Autodesk Inventor part; units mm, degrees
(part 7 of 15)
  arc A2930 (57.5832, 42.092) -> (57.6848, 42.092) centre (57.634, 42.092) ccw
  line L1321 (60.642, 43.084) -> (60.642, 45.116)
  arc A2931 (60.6928, 45.116) -> (60.5912, 45.116) centre (60.642, 45.116) ccw
  arc A2932 (60.5912, 43.084) -> (60.6928, 43.084) centre (60.642, 43.084) ccw
  line L1322 (60.642, 45.116) -> (61.658, 45.116)
  arc A2933 (61.658, 45.0652) -> (61.658, 45.1668) centre (61.658, 45.116) ccw
  arc A2934 (60.642, 45.1668) -> (60.642, 45.0652) centre (60.642, 45.116) ccw
  line L1323 (61.658, 45.116) -> (61.658, 43.084)
  arc A2935 (61.6072, 43.084) -> (61.7088, 43.084) centre (61.658, 43.084) ccw
  arc A2936 (61.7088, 45.116) -> (61.6072, 45.116) centre (61.658, 45.116) ccw
  line L1324 (61.658, 43.084) -> (60.642, 43.084)
  arc A2937 (60.642, 43.1348) -> (60.642, 43.0332) centre (60.642, 43.084) ccw
  arc A2938 (61.658, 43.0332) -> (61.658, 43.1348) centre (61.658, 43.084) ccw
  line L1325 (55.658, 51.116) -> (55.658, 49.084)
  arc A2939 (55.6072, 49.084) -> (55.7088, 49.084) centre (55.658, 49.084) ccw
  arc A2940 (55.7088, 51.116) -> (55.6072, 51.116) centre (55.658, 51.116) ccw
  line L1326 (55.658, 49.084) -> (54.642, 49.084)
  arc A2941 (54.642, 49.1348) -> (54.642, 49.0332) centre (54.642, 49.084) ccw
  arc A2942 (55.658, 49.0332) -> (55.658, 49.1348) centre (55.658, 49.084) ccw
  line L1327 (54.642, 49.084) -> (54.642, 51.116)
  arc A2943 (54.6928, 51.116) -> (54.5912, 51.116) centre (54.642, 51.116) ccw
  arc A2944 (54.5912, 49.084) -> (54.6928, 49.084) centre (54.642, 49.084) ccw
  line L1328 (54.642, 51.116) -> (55.658, 51.116)
  arc A2945 (55.658, 51.0652) -> (55.658, 51.1668) centre (55.658, 51.116) ccw
  arc A2946 (54.642, 51.1668) -> (54.642, 51.0652) centre (54.642, 51.116) ccw
  line L1329 (61.166, 33.892) -> (59.134, 33.892)
  arc A2947 (59.134, 33.9428) -> (59.134, 33.8412) centre (59.134, 33.892) ccw
  arc A2948 (61.166, 33.8412) -> (61.166, 33.9428) centre (61.166, 33.892) ccw
  line L1330 (59.134, 33.892) -> (59.134, 34.908)
  arc A2949 (59.1848, 34.908) -> (59.0832, 34.908) centre (59.134, 34.908) ccw
  arc A2950 (59.0832, 33.892) -> (59.1848, 33.892) centre (59.134, 33.892) ccw
  line L1331 (59.134, 34.908) -> (61.166, 34.908)
  arc A2951 (61.166, 34.8572) -> (61.166, 34.9588) centre (61.166, 34.908) ccw
  arc A2952 (59.134, 34.9588) -> (59.134, 34.8572) centre (59.134, 34.908) ccw
  line L1332 (61.166, 34.908) -> (61.166, 33.892)
  arc A2953 (61.1152, 33.892) -> (61.2168, 33.892) centre (61.166, 33.892) ccw
  arc A2954 (61.2168, 34.908) -> (61.1152, 34.908) centre (61.166, 34.908) ccw
  line L1333 (63.166, 33.892) -> (61.134, 33.892)
  arc A2955 (61.134, 33.9428) -> (61.134, 33.8412) centre (61.134, 33.892) ccw
  arc A2956 (63.166, 33.8412) -> (63.166, 33.9428) centre (63.166, 33.892) ccw
  line L1334 (61.134, 33.892) -> (61.134, 34.908)
  arc A2957 (61.1848, 34.908) -> (61.0832, 34.908) centre (61.134, 34.908) ccw
  arc A2958 (61.0832, 33.892) -> (61.1848, 33.892) centre (61.134, 33.892) ccw
  line L1335 (61.134, 34.908) -> (63.166, 34.908)
  arc A2959 (63.166, 34.8572) -> (63.166, 34.9588) centre (63.166, 34.908) ccw
  arc A2960 (61.134, 34.9588) -> (61.134, 34.8572) centre (61.134, 34.908) ccw
  line L1336 (63.166, 34.908) -> (63.166, 33.892)
  arc A2961 (63.1152, 33.892) -> (63.2168, 33.892) centre (63.166, 33.892) ccw
  arc A2962 (63.2168, 34.908) -> (63.1152, 34.908) centre (63.166, 34.908) ccw
  line L1337 (52.658, 43.116) -> (52.658, 41.084)
  arc A2963 (52.6072, 41.084) -> (52.7088, 41.084) centre (52.658, 41.084) ccw
  arc A2964 (52.7088, 43.116) -> (52.6072, 43.116) centre (52.658, 43.116) ccw
  line L1338 (52.658, 41.084) -> (51.642, 41.084)
  arc A2965 (51.642, 41.1348) -> (51.642, 41.0332) centre (51.642, 41.084) ccw
  arc A2966 (52.658, 41.0332) -> (52.658, 41.1348) centre (52.658, 41.084) ccw
  line L1339 (51.642, 41.084) -> (51.642, 43.116)
  arc A2967 (51.6928, 43.116) -> (51.5912, 43.116) centre (51.642, 43.116) ccw
  arc A2968 (51.5912, 41.084) -> (51.6928, 41.084) centre (51.642, 41.084) ccw
  line L1340 (51.642, 43.116) -> (52.658, 43.116)
  arc A2969 (52.658, 43.0652) -> (52.658, 43.1668) centre (52.658, 43.116) ccw
  arc A2970 (51.642, 43.1668) -> (51.642, 43.0652) centre (51.642, 43.116) ccw
  line L1341 (51.666, 42.092) -> (49.634, 42.092)
  arc A2971 (49.634, 42.1428) -> (49.634, 42.0412) centre (49.634, 42.092) ccw
  arc A2972 (51.666, 42.0412) -> (51.666, 42.1428) centre (51.666, 42.092) ccw
  line L1342 (49.634, 42.092) -> (49.634, 43.108)
  arc A2973 (49.6848, 43.108) -> (49.5832, 43.108) centre (49.634, 43.108) ccw
  arc A2974 (49.5832, 42.092) -> (49.6848, 42.092) centre (49.634, 42.092) ccw
  line L1343 (49.634, 43.108) -> (51.666, 43.108)
  arc A2975 (51.666, 43.0572) -> (51.666, 43.1588) centre (51.666, 43.108) ccw
  arc A2976 (49.634, 43.1588) -> (49.634, 43.0572) centre (49.634, 43.108) ccw
  line L1344 (51.666, 43.108) -> (51.666, 42.092)
  arc A2977 (51.6152, 42.092) -> (51.7168, 42.092) centre (51.666, 42.092) ccw
  arc A2978 (51.7168, 43.108) -> (51.6152, 43.108) centre (51.666, 43.108) ccw
  line L1345 (51.634, 49.108) -> (53.666, 49.108)
  arc A2979 (53.666, 49.0572) -> (53.666, 49.1588) centre (53.666, 49.108) ccw
  arc A2980 (51.634, 49.1588) -> (51.634, 49.0572) centre (51.634, 49.108) ccw
  line L1346 (53.666, 49.108) -> (53.666, 48.092)
  arc A2981 (53.6152, 48.092) -> (53.7168, 48.092) centre (53.666, 48.092) ccw
  arc A2982 (53.7168, 49.108) -> (53.6152, 49.108) centre (53.666, 49.108) ccw
  line L1347 (53.666, 48.092) -> (51.634, 48.092)
  arc A2983 (51.634, 48.1428) -> (51.634, 48.0412) centre (51.634, 48.092) ccw
  arc A2984 (53.666, 48.0412) -> (53.666, 48.1428) centre (53.666, 48.092) ccw
  line L1348 (51.634, 48.092) -> (51.634, 49.108)
  arc A2985 (51.6848, 49.108) -> (51.5832, 49.108) centre (51.634, 49.108) ccw
  arc A2986 (51.5832, 48.092) -> (51.6848, 48.092) centre (51.634, 48.092) ccw
  line L1349 (51.634, 44.108) -> (53.666, 44.108)
  arc A2987 (53.666, 44.0572) -> (53.666, 44.1588) centre (53.666, 44.108) ccw
  arc A2988 (51.634, 44.1588) -> (51.634, 44.0572) centre (51.634, 44.108) ccw
  line L1350 (53.666, 44.108) -> (53.666, 43.092)
  arc A2989 (53.6152, 43.092) -> (53.7168, 43.092) centre (53.666, 43.092) ccw
  arc A2990 (53.7168, 44.108) -> (53.6152, 44.108) centre (53.666, 44.108) ccw
  line L1351 (53.666, 43.092) -> (51.634, 43.092)
  arc A2991 (51.634, 43.1428) -> (51.634, 43.0412) centre (51.634, 43.092) ccw
  arc A2992 (53.666, 43.0412) -> (53.666, 43.1428) centre (53.666, 43.092) ccw
  line L1352 (51.634, 43.092) -> (51.634, 44.108)
  arc A2993 (51.6848, 44.108) -> (51.5832, 44.108) centre (51.634, 44.108) ccw
  arc A2994 (51.5832, 43.092) -> (51.6848, 43.092) centre (51.634, 43.092) ccw
  line L1353 (51.634, 45.108) -> (53.666, 45.108)
  arc A2995 (53.666, 45.0572) -> (53.666, 45.1588) centre (53.666, 45.108) ccw
  arc A2996 (51.634, 45.1588) -> (51.634, 45.0572) centre (51.634, 45.108) ccw
  line L1354 (53.666, 45.108) -> (53.666, 44.092)
  arc A2997 (53.6152, 44.092) -> (53.7168, 44.092) centre (53.666, 44.092) ccw
  arc A2998 (53.7168, 45.108) -> (53.6152, 45.108) centre (53.666, 45.108) ccw
  line L1355 (53.666, 44.092) -> (51.634, 44.092)
  arc A2999 (51.634, 44.1428) -> (51.634, 44.0412) centre (51.634, 44.092) ccw
  arc A3000 (53.666, 44.0412) -> (53.666, 44.1428) centre (53.666, 44.092) ccw
  line L1356 (51.634, 44.092) -> (51.634, 45.108)
  arc A3001 (51.6848, 45.108) -> (51.5832, 45.108) centre (51.634, 45.108) ccw
  arc A3002 (51.5832, 44.092) -> (51.6848, 44.092) centre (51.634, 44.092) ccw
  line L1357 (67.958, 53.716) -> (67.958, 51.684)
  arc A3003 (67.9072, 51.684) -> (68.0088, 51.684) centre (67.958, 51.684) ccw
  arc A3004 (68.0088, 53.716) -> (67.9072, 53.716) centre (67.958, 53.716) ccw
  line L1358 (67.958, 51.684) -> (66.942, 51.684)
  arc A3005 (66.942, 51.7348) -> (66.942, 51.6332) centre (66.942, 51.684) ccw
  arc A3006 (67.958, 51.6332) -> (67.958, 51.7348) centre (67.958, 51.684) ccw
  line L1359 (66.942, 51.684) -> (66.942, 53.716)
  arc A3007 (66.9928, 53.716) -> (66.8912, 53.716) centre (66.942, 53.716) ccw
  arc A3008 (66.8912, 51.684) -> (66.9928, 51.684) centre (66.942, 51.684) ccw
  line L1360 (66.942, 53.716) -> (67.958, 53.716)
  arc A3009 (67.958, 53.6652) -> (67.958, 53.7668) centre (67.958, 53.716) ccw
  arc A3010 (66.942, 53.7668) -> (66.942, 53.6652) centre (66.942, 53.716) ccw
  line L1361 (61.442, 51.684) -> (61.442, 53.716)
  arc A3011 (61.4928, 53.716) -> (61.3912, 53.716) centre (61.442, 53.716) ccw
  arc A3012 (61.3912, 51.684) -> (61.4928, 51.684) centre (61.442, 51.684) ccw
  line L1362 (61.442, 53.716) -> (62.458, 53.716)
  arc A3013 (62.458, 53.6652) -> (62.458, 53.7668) centre (62.458, 53.716) ccw
  arc A3014 (61.442, 53.7668) -> (61.442, 53.6652) centre (61.442, 53.716) ccw
  line L1363 (62.458, 53.716) -> (62.458, 51.684)
  arc A3015 (62.4072, 51.684) -> (62.5088, 51.684) centre (62.458, 51.684) ccw
  arc A3016 (62.5088, 53.716) -> (62.4072, 53.716) centre (62.458, 53.716) ccw
  line L1364 (62.458, 51.684) -> (61.442, 51.684)
  arc A3017 (61.442, 51.7348) -> (61.442, 51.6332) centre (61.442, 51.684) ccw
  arc A3018 (62.458, 51.6332) -> (62.458, 51.7348) centre (62.458, 51.684) ccw
  line L1365 (-2.616, 56.708) -> (-0.584, 56.708)
  arc A3019 (-0.584, 56.6572) -> (-0.584, 56.7588) centre (-0.584, 56.708) ccw
  arc A3020 (-2.616, 56.7588) -> (-2.616, 56.6572) centre (-2.616, 56.708) ccw
  line L1366 (-0.584, 56.708) -> (-0.584, 55.692)
  arc A3021 (-0.6348, 55.692) -> (-0.5332, 55.692) centre (-0.584, 55.692) ccw
  arc A3022 (-0.5332, 56.708) -> (-0.6348, 56.708) centre (-0.584, 56.708) ccw
  line L1367 (-0.584, 55.692) -> (-2.616, 55.692)
  arc A3023 (-2.616, 55.7428) -> (-2.616, 55.6412) centre (-2.616, 55.692) ccw
  arc A3024 (-0.584, 55.6412) -> (-0.584, 55.7428) centre (-0.584, 55.692) ccw
  line L1368 (-2.616, 55.692) -> (-2.616, 56.708)
  arc A3025 (-2.5652, 56.708) -> (-2.6668, 56.708) centre (-2.616, 56.708) ccw
  arc A3026 (-2.6668, 55.692) -> (-2.5652, 55.692) centre (-2.616, 55.692) ccw
  line L1369 (-0.584, 51.692) -> (-2.616, 51.692)
  arc A3027 (-2.616, 51.7428) -> (-2.616, 51.6412) centre (-2.616, 51.692) ccw
  arc A3028 (-0.584, 51.6412) -> (-0.584, 51.7428) centre (-0.584, 51.692) ccw
  line L1370 (-2.616, 51.692) -> (-2.616, 52.708)
  arc A3029 (-2.5652, 52.708) -> (-2.6668, 52.708) centre (-2.616, 52.708) ccw
  arc A3030 (-2.6668, 51.692) -> (-2.5652, 51.692) centre (-2.616, 51.692) ccw
  line L1371 (-2.616, 52.708) -> (-0.584, 52.708)
  arc A3031 (-0.584, 52.6572) -> (-0.584, 52.7588) centre (-0.584, 52.708) ccw
  arc A3032 (-2.616, 52.7588) -> (-2.616, 52.6572) centre (-2.616, 52.708) ccw
  line L1372 (-0.584, 52.708) -> (-0.584, 51.692)
  arc A3033 (-0.6348, 51.692) -> (-0.5332, 51.692) centre (-0.584, 51.692) ccw
  arc A3034 (-0.5332, 52.708) -> (-0.6348, 52.708) centre (-0.584, 52.708) ccw
  line L1373 (-2.616, 53.708) -> (-0.584, 53.708)
  arc A3035 (-0.584, 53.6572) -> (-0.584, 53.7588) centre (-0.584, 53.708) ccw
  arc A3036 (-2.616, 53.7588) -> (-2.616, 53.6572) centre (-2.616, 53.708) ccw
  line L1374 (-0.584, 53.708) -> (-0.584, 52.692)
  arc A3037 (-0.6348, 52.692) -> (-0.5332, 52.692) centre (-0.584, 52.692) ccw
  arc A3038 (-0.5332, 53.708) -> (-0.6348, 53.708) centre (-0.584, 53.708) ccw
  line L1375 (-0.584, 52.692) -> (-2.616, 52.692)
  arc A3039 (-2.616, 52.7428) -> (-2.616, 52.6412) centre (-2.616, 52.692) ccw
  arc A3040 (-0.584, 52.6412) -> (-0.584, 52.7428) centre (-0.584, 52.692) ccw
  line L1376 (-2.616, 52.692) -> (-2.616, 53.708)
  arc A3041 (-2.5652, 53.708) -> (-2.6668, 53.708) centre (-2.616, 53.708) ccw
  arc A3042 (-2.6668, 52.692) -> (-2.5652, 52.692) centre (-2.616, 52.692) ccw
  line L1377 (-2.616, 54.708) -> (-0.584, 54.708)
  arc A3043 (-0.584, 54.6572) -> (-0.584, 54.7588) centre (-0.584, 54.708) ccw
  arc A3044 (-2.616, 54.7588) -> (-2.616, 54.6572) centre (-2.616, 54.708) ccw
  line L1378 (-0.584, 54.708) -> (-0.584, 53.692)
  arc A3045 (-0.6348, 53.692) -> (-0.5332, 53.692) centre (-0.584, 53.692) ccw
  arc A3046 (-0.5332, 54.708) -> (-0.6348, 54.708) centre (-0.584, 54.708) ccw
  line L1379 (-0.584, 53.692) -> (-2.616, 53.692)
  arc A3047 (-2.616, 53.7428) -> (-2.616, 53.6412) centre (-2.616, 53.692) ccw
  arc A3048 (-0.584, 53.6412) -> (-0.584, 53.7428) centre (-0.584, 53.692) ccw
  line L1380 (-2.616, 53.692) -> (-2.616, 54.708)
  arc A3049 (-2.5652, 54.708) -> (-2.6668, 54.708) centre (-2.616, 54.708) ccw
  arc A3050 (-2.6668, 53.692) -> (-2.5652, 53.692) centre (-2.616, 53.692) ccw
  line L1381 (-2.608, 50.684) -> (-2.608, 52.716)
  arc A3051 (-2.5572, 52.716) -> (-2.6588, 52.716) centre (-2.608, 52.716) ccw
  arc A3052 (-2.6588, 50.684) -> (-2.5572, 50.684) centre (-2.608, 50.684) ccw
  line L1382 (-2.608, 52.716) -> (-1.592, 52.716)
  arc A3053 (-1.592, 52.6652) -> (-1.592, 52.7668) centre (-1.592, 52.716) ccw
  arc A3054 (-2.608, 52.7668) -> (-2.608, 52.6652) centre (-2.608, 52.716) ccw
  line L1383 (-1.592, 52.716) -> (-1.592, 50.684)
  arc A3055 (-1.6428, 50.684) -> (-1.5412, 50.684) centre (-1.592, 50.684) ccw
  arc A3056 (-1.5412, 52.716) -> (-1.6428, 52.716) centre (-1.592, 52.716) ccw
  line L1384 (-1.592, 50.684) -> (-2.608, 50.684)
  arc A3057 (-2.608, 50.7348) -> (-2.608, 50.6332) centre (-2.608, 50.684) ccw
  arc A3058 (-1.592, 50.6332) -> (-1.592, 50.7348) centre (-1.592, 50.684) ccw
  line L1385 (1.292, 39.784) -> (1.292, 41.816)
  arc A3059 (1.3428, 41.816) -> (1.2412, 41.816) centre (1.292, 41.816) ccw
  arc A3060 (1.2412, 39.784) -> (1.3428, 39.784) centre (1.292, 39.784) ccw
  line L1386 (1.292, 41.816) -> (2.308, 41.816)
  arc A3061 (2.308, 41.7652) -> (2.308, 41.8668) centre (2.308, 41.816) ccw
  arc A3062 (1.292, 41.8668) -> (1.292, 41.7652) centre (1.292, 41.816) ccw
  line L1387 (2.308, 41.816) -> (2.308, 39.784)
  arc A3063 (2.2572, 39.784) -> (2.3588, 39.784) centre (2.308, 39.784) ccw
  arc A3064 (2.3588, 41.816) -> (2.2572, 41.816) centre (2.308, 41.816) ccw
  line L1388 (2.308, 39.784) -> (1.292, 39.784)
  arc A3065 (1.292, 39.8348) -> (1.292, 39.7332) centre (1.292, 39.784) ccw
  arc A3066 (2.308, 39.7332) -> (2.308, 39.8348) centre (2.308, 39.784) ccw
  line L1389 (14.684, 22.208) -> (16.716, 22.208)
  arc A3067 (16.716, 22.1572) -> (16.716, 22.2588) centre (16.716, 22.208) ccw
  arc A3068 (14.684, 22.2588) -> (14.684, 22.1572) centre (14.684, 22.208) ccw
  line L1390 (16.716, 22.208) -> (16.716, 21.192)
  arc A3069 (16.6652, 21.192) -> (16.7668, 21.192) centre (16.716, 21.192) ccw
  arc A3070 (16.7668, 22.208) -> (16.6652, 22.208) centre (16.716, 22.208) ccw
  line L1391 (16.716, 21.192) -> (14.684, 21.192)
  arc A3071 (14.684, 21.2428) -> (14.684, 21.1412) centre (14.684, 21.192) ccw
  arc A3072 (16.716, 21.1412) -> (16.716, 21.2428) centre (16.716, 21.192) ccw
  line L1392 (14.684, 21.192) -> (14.684, 22.208)
  arc A3073 (14.7348, 22.208) -> (14.6332, 22.208) centre (14.684, 22.208) ccw
  arc A3074 (14.6332, 21.192) -> (14.7348, 21.192) centre (14.684, 21.192) ccw
  line L1393 (20.916, 21.192) -> (18.884, 21.192)
  arc A3075 (18.884, 21.2428) -> (18.884, 21.1412) centre (18.884, 21.192) ccw
  arc A3076 (20.916, 21.1412) -> (20.916, 21.2428) centre (20.916, 21.192) ccw
  line L1394 (18.884, 21.192) -> (18.884, 22.208)
  arc A3077 (18.9348, 22.208) -> (18.8332, 22.208) centre (18.884, 22.208) ccw
  arc A3078 (18.8332, 21.192) -> (18.9348, 21.192) centre (18.884, 21.192) ccw
  line L1395 (18.884, 22.208) -> (20.916, 22.208)
  arc A3079 (20.916, 22.1572) -> (20.916, 22.2588) centre (20.916, 22.208) ccw
  arc A3080 (18.884, 22.2588) -> (18.884, 22.1572) centre (18.884, 22.208) ccw
  line L1396 (20.916, 22.208) -> (20.916, 21.192)
  arc A3081 (20.8652, 21.192) -> (20.9668, 21.192) centre (20.916, 21.192) ccw
  arc A3082 (20.9668, 22.208) -> (20.8652, 22.208) centre (20.916, 22.208) ccw
  line L1397 (12.684, 22.208) -> (14.716, 22.208)
  arc A3083 (14.716, 22.1572) -> (14.716, 22.2588) centre (14.716, 22.208) ccw
  arc A3084 (12.684, 22.2588) -> (12.684, 22.1572) centre (12.684, 22.208) ccw
  line L1398 (14.716, 22.208) -> (14.716, 21.192)
  arc A3085 (14.6652, 21.192) -> (14.7668, 21.192) centre (14.716, 21.192) ccw
  arc A3086 (14.7668, 22.208) -> (14.6652, 22.208) centre (14.716, 22.208) ccw
  line L1399 (14.716, 21.192) -> (12.684, 21.192)
  arc A3087 (12.684, 21.2428) -> (12.684, 21.1412) centre (12.684, 21.192) ccw
  arc A3088 (14.716, 21.1412) -> (14.716, 21.2428) centre (14.716, 21.192) ccw
  line L1400 (12.684, 21.192) -> (12.684, 22.208)
  arc A3089 (12.7348, 22.208) -> (12.6332, 22.208) centre (12.684, 22.208) ccw
  arc A3090 (12.6332, 21.192) -> (12.7348, 21.192) centre (12.684, 21.192) ccw
  line L1401 (14.684, 11.808) -> (16.716, 11.808)
  arc A3091 (16.716, 11.7572) -> (16.716, 11.8588) centre (16.716, 11.808) ccw
  arc A3092 (14.684, 11.8588) -> (14.684, 11.7572) centre (14.684, 11.808) ccw
  line L1402 (16.716, 11.808) -> (16.716, 10.792)
  arc A3093 (16.6652, 10.792) -> (16.7668, 10.792) centre (16.716, 10.792) ccw
  arc A3094 (16.7668, 11.808) -> (16.6652, 11.808) centre (16.716, 11.808) ccw
  line L1403 (16.716, 10.792) -> (14.684, 10.792)
  arc A3095 (14.684, 10.8428) -> (14.684, 10.7412) centre (14.684, 10.792) ccw
  arc A3096 (16.716, 10.7412) -> (16.716, 10.8428) centre (16.716, 10.792) ccw
  line L1404 (14.684, 10.792) -> (14.684, 11.808)
  arc A3097 (14.7348, 11.808) -> (14.6332, 11.808) centre (14.684, 11.808) ccw
  arc A3098 (14.6332, 10.792) -> (14.7348, 10.792) centre (14.684, 10.792) ccw
  line L1405 (20.916, 10.792) -> (18.884, 10.792)
  arc A3099 (18.884, 10.8428) -> (18.884, 10.7412) centre (18.884, 10.792) ccw
  arc A3100 (20.916, 10.7412) -> (20.916, 10.8428) centre (20.916, 10.792) ccw
  line L1406 (18.884, 10.792) -> (18.884, 11.808)
  arc A3101 (18.9348, 11.808) -> (18.8332, 11.808) centre (18.884, 11.808) ccw
  arc A3102 (18.8332, 10.792) -> (18.9348, 10.792) centre (18.884, 10.792) ccw
  line L1407 (18.884, 11.808) -> (20.916, 11.808)
  arc A3103 (20.916, 11.7572) -> (20.916, 11.8588) centre (20.916, 11.808) ccw
  arc A3104 (18.884, 11.8588) -> (18.884, 11.7572) centre (18.884, 11.808) ccw
  line L1408 (20.916, 11.808) -> (20.916, 10.792)
  arc A3105 (20.8652, 10.792) -> (20.9668, 10.792) centre (20.916, 10.792) ccw
  arc A3106 (20.9668, 11.808) -> (20.8652, 11.808) centre (20.916, 11.808) ccw
  line L1409 (22.884, -9.992) -> (24.916, -9.992)
  arc A3107 (24.916, -10.0428) -> (24.916, -9.9412) centre (24.916, -9.992) ccw
  arc A3108 (22.884, -9.9412) -> (22.884, -10.0428) centre (22.884, -9.992) ccw
  line L1410 (24.916, -9.992) -> (24.916, -11.008)
  arc A3109 (24.8652, -11.008) -> (24.9668, -11.008) centre (24.916, -11.008) ccw
  arc A3110 (24.9668, -9.992) -> (24.8652, -9.992) centre (24.916, -9.992) ccw
  line L1411 (24.916, -11.008) -> (22.884, -11.008)
  arc A3111 (22.884, -10.9572) -> (22.884, -11.0588) centre (22.884, -11.008) ccw
  arc A3112 (24.916, -11.0588) -> (24.916, -10.9572) centre (24.916, -11.008) ccw
  line L1412 (22.884, -11.008) -> (22.884, -9.992)
  arc A3113 (22.9348, -9.992) -> (22.8332, -9.992) centre (22.884, -9.992) ccw
  arc A3114 (22.8332, -11.008) -> (22.9348, -11.008) centre (22.884, -11.008) ccw
  line L1413 (16.684, 11.808) -> (18.716, 11.808)
  arc A3115 (18.716, 11.7572) -> (18.716, 11.8588) centre (18.716, 11.808) ccw
  arc A3116 (16.684, 11.8588) -> (16.684, 11.7572) centre (16.684, 11.808) ccw
  line L1414 (18.716, 11.808) -> (18.716, 10.792)
  arc A3117 (18.6652, 10.792) -> (18.7668, 10.792) centre (18.716, 10.792) ccw
  arc A3118 (18.7668, 11.808) -> (18.6652, 11.808) centre (18.716, 11.808) ccw
  line L1415 (18.716, 10.792) -> (16.684, 10.792)
  arc A3119 (16.684, 10.8428) -> (16.684, 10.7412) centre (16.684, 10.792) ccw
  arc A3120 (18.716, 10.7412) -> (18.716, 10.8428) centre (18.716, 10.792) ccw
  line L1416 (16.684, 10.792) -> (16.684, 11.808)
  arc A3121 (16.7348, 11.808) -> (16.6332, 11.808) centre (16.684, 11.808) ccw
  arc A3122 (16.6332, 10.792) -> (16.7348, 10.792) centre (16.684, 10.792) ccw
  line L1417 (18.684, -13.992) -> (20.716, -13.992)
  arc A3123 (20.716, -14.0428) -> (20.716, -13.9412) centre (20.716, -13.992) ccw
  arc A3124 (18.684, -13.9412) -> (18.684, -14.0428) centre (18.684, -13.992) ccw
  line L1418 (20.716, -13.992) -> (20.716, -15.008)
  arc A3125 (20.6652, -15.008) -> (20.7668, -15.008) centre (20.716, -15.008) ccw
  arc A3126 (20.7668, -13.992) -> (20.6652, -13.992) centre (20.716, -13.992) ccw
  line L1419 (20.716, -15.008) -> (18.684, -15.008)
  arc A3127 (18.684, -14.9572) -> (18.684, -15.0588) centre (18.684, -15.008) ccw
  arc A3128 (20.716, -15.0588) -> (20.716, -14.9572) centre (20.716, -15.008) ccw
  line L1420 (18.684, -15.008) -> (18.684, -13.992)
  arc A3129 (18.7348, -13.992) -> (18.6332, -13.992) centre (18.684, -13.992) ccw
  arc A3130 (18.6332, -15.008) -> (18.7348, -15.008) centre (18.684, -15.008) ccw
  line L1421 (18.716, 5.692) -> (16.684, 5.692)
  arc A3131 (16.684, 5.7428) -> (16.684, 5.6412) centre (16.684, 5.692) ccw
  arc A3132 (18.716, 5.6412) -> (18.716, 5.7428) centre (18.716, 5.692) ccw
  line L1422 (16.684, 5.692) -> (16.684, 6.708)
  arc A3133 (16.7348, 6.708) -> (16.6332, 6.708) centre (16.684, 6.708) ccw
  arc A3134 (16.6332, 5.692) -> (16.7348, 5.692) centre (16.684, 5.692) ccw
  line L1423 (16.684, 6.708) -> (18.716, 6.708)
  arc A3135 (18.716, 6.6572) -> (18.716, 6.7588) centre (18.716, 6.708) ccw
  arc A3136 (16.684, 6.7588) -> (16.684, 6.6572) centre (16.684, 6.708) ccw
  line L1424 (18.716, 6.708) -> (18.716, 5.692)
  arc A3137 (18.6652, 5.692) -> (18.7668, 5.692) centre (18.716, 5.692) ccw
  arc A3138 (18.7668, 6.708) -> (18.6652, 6.708) centre (18.716, 6.708) ccw
  line L1425 (12.684, -8.992) -> (14.716, -8.992)
  arc A3139 (14.716, -9.0428) -> (14.716, -8.9412) centre (14.716, -8.992) ccw
  arc A3140 (12.684, -8.9412) -> (12.684, -9.0428) centre (12.684, -8.992) ccw
  line L1426 (14.716, -8.992) -> (14.716, -10.008)
  arc A3141 (14.6652, -10.008) -> (14.7668, -10.008) centre (14.716, -10.008) ccw
  arc A3142 (14.7668, -8.992) -> (14.6652, -8.992) centre (14.716, -8.992) ccw
  line L1427 (14.716, -10.008) -> (12.684, -10.008)
  arc A3143 (12.684, -9.9572) -> (12.684, -10.0588) centre (12.684, -10.008) ccw
  arc A3144 (14.716, -10.0588) -> (14.716, -9.9572) centre (14.716, -10.008) ccw
  line L1428 (12.684, -10.008) -> (12.684, -8.992)
  arc A3145 (12.7348, -8.992) -> (12.6332, -8.992) centre (12.684, -8.992) ccw
  arc A3146 (12.6332, -10.008) -> (12.7348, -10.008) centre (12.684, -10.008) ccw
  line L1429 (12.684, 11.808) -> (14.716, 11.808)
  arc A3147 (14.716, 11.7572) -> (14.716, 11.8588) centre (14.716, 11.808) ccw
  arc A3148 (12.684, 11.8588) -> (12.684, 11.7572) centre (12.684, 11.808) ccw
  line L1430 (14.716, 11.808) -> (14.716, 10.792)
  arc A3149 (14.6652, 10.792) -> (14.7668, 10.792) centre (14.716, 10.792) ccw
  arc A3150 (14.7668, 11.808) -> (14.6652, 11.808) centre (14.716, 11.808) ccw
  line L1431 (14.716, 10.792) -> (12.684, 10.792)
  arc A3151 (12.684, 10.8428) -> (12.684, 10.7412) centre (12.684, 10.792) ccw
  arc A3152 (14.716, 10.7412) -> (14.716, 10.8428) centre (14.716, 10.792) ccw
  line L1432 (12.684, 10.792) -> (12.684, 11.808)
  arc A3153 (12.7348, 11.808) -> (12.6332, 11.808) centre (12.684, 11.808) ccw
  arc A3154 (12.6332, 10.792) -> (12.7348, 10.792) centre (12.684, 10.792) ccw
  line L1433 (14.684, 1.408) -> (16.716, 1.408)
  arc A3155 (16.716, 1.3572) -> (16.716, 1.4588) centre (16.716, 1.408) ccw
  arc A3156 (14.684, 1.4588) -> (14.684, 1.3572) centre (14.684, 1.408) ccw
  line L1434 (16.716, 1.408) -> (16.716, 0.392)
  arc A3157 (16.6652, 0.392) -> (16.7668, 0.392) centre (16.716, 0.392) ccw
  arc A3158 (16.7668, 1.408) -> (16.6652, 1.408) centre (16.716, 1.408) ccw
  line L1435 (16.716, 0.392) -> (14.684, 0.392)
  arc A3159 (14.684, 0.4428) -> (14.684, 0.3412) centre (14.684, 0.392) ccw
  arc A3160 (16.716, 0.3412) -> (16.716, 0.4428) centre (16.716, 0.392) ccw
  line L1436 (14.684, 0.392) -> (14.684, 1.408)
  arc A3161 (14.7348, 1.408) -> (14.6332, 1.408) centre (14.684, 1.408) ccw
  arc A3162 (14.6332, 0.392) -> (14.7348, 0.392) centre (14.684, 0.392) ccw
  line L1437 (20.916, 0.392) -> (18.884, 0.392)
  arc A3163 (18.884, 0.4428) -> (18.884, 0.3412) centre (18.884, 0.392) ccw
  arc A3164 (20.916, 0.3412) -> (20.916, 0.4428) centre (20.916, 0.392) ccw
  line L1438 (18.884, 0.392) -> (18.884, 1.408)
  arc A3165 (18.9348, 1.408) -> (18.8332, 1.408) centre (18.884, 1.408) ccw
  arc A3166 (18.8332, 0.392) -> (18.9348, 0.392) centre (18.884, 0.392) ccw
  line L1439 (18.884, 1.408) -> (20.916, 1.408)
  arc A3167 (20.916, 1.3572) -> (20.916, 1.4588) centre (20.916, 1.408) ccw
  arc A3168 (18.884, 1.4588) -> (18.884, 1.3572) centre (18.884, 1.408) ccw
  line L1440 (20.916, 1.408) -> (20.916, 0.392)
  arc A3169 (20.8652, 0.392) -> (20.9668, 0.392) centre (20.916, 0.392) ccw
  arc A3170 (20.9668, 1.408) -> (20.8652, 1.408) centre (20.916, 1.408) ccw
  line L1441 (16.684, 1.408) -> (18.716, 1.408)
  arc A3171 (18.716, 1.3572) -> (18.716, 1.4588) centre (18.716, 1.408) ccw
  arc A3172 (16.684, 1.4588) -> (16.684, 1.3572) centre (16.684, 1.408) ccw
  line L1442 (18.716, 1.408) -> (18.716, 0.392)
  arc A3173 (18.6652, 0.392) -> (18.7668, 0.392) centre (18.716, 0.392) ccw
  arc A3174 (18.7668, 1.408) -> (18.6652, 1.408) centre (18.716, 1.408) ccw
  line L1443 (18.716, 0.392) -> (16.684, 0.392)
  arc A3175 (16.684, 0.4428) -> (16.684, 0.3412) centre (16.684, 0.392) ccw
  arc A3176 (18.716, 0.3412) -> (18.716, 0.4428) centre (18.716, 0.392) ccw
  line L1444 (16.684, 0.392) -> (16.684, 1.408)
  arc A3177 (16.7348, 1.408) -> (16.6332, 1.408) centre (16.684, 1.408) ccw
  arc A3178 (16.6332, 0.392) -> (16.7348, 0.392) centre (16.684, 0.392) ccw
  line L1445 (18.916, -4.608) -> (16.884, -4.608)
  arc A3179 (16.884, -4.5572) -> (16.884, -4.6588) centre (16.884, -4.608) ccw
  arc A3180 (18.916, -4.6588) -> (18.916, -4.5572) centre (18.916, -4.608) ccw
  line L1446 (16.884, -4.608) -> (16.884, -3.592)
  arc A3181 (16.9348, -3.592) -> (16.8332, -3.592) centre (16.884, -3.592) ccw
  arc A3182 (16.8332, -4.608) -> (16.9348, -4.608) centre (16.884, -4.608) ccw
  line L1447 (16.884, -3.592) -> (18.916, -3.592)
  arc A3183 (18.916, -3.6428) -> (18.916, -3.5412) centre (18.916, -3.592) ccw
  arc A3184 (16.884, -3.5412) -> (16.884, -3.6428) centre (16.884, -3.592) ccw
  line L1448 (18.916, -3.592) -> (18.916, -4.608)
  arc A3185 (18.8652, -4.608) -> (18.9668, -4.608) centre (18.916, -4.608) ccw
  arc A3186 (18.9668, -3.592) -> (18.8652, -3.592) centre (18.916, -3.592) ccw
  line L1449 (12.684, 1.408) -> (14.716, 1.408)
  arc A3187 (14.716, 1.3572) -> (14.716, 1.4588) centre (14.716, 1.408) ccw
  arc A3188 (12.684, 1.4588) -> (12.684, 1.3572) centre (12.684, 1.408) ccw
  line L1450 (14.716, 1.408) -> (14.716, 0.392)
  arc A3189 (14.6652, 0.392) -> (14.7668, 0.392) centre (14.716, 0.392) ccw
  arc A3190 (14.7668, 1.408) -> (14.6652, 1.408) centre (14.716, 1.408) ccw
  line L1451 (14.716, 0.392) -> (12.684, 0.392)
  arc A3191 (12.684, 0.4428) -> (12.684, 0.3412) centre (12.684, 0.392) ccw
  arc A3192 (14.716, 0.3412) -> (14.716, 0.4428) centre (14.716, 0.392) ccw
  line L1452 (12.684, 0.392) -> (12.684, 1.408)
  arc A3193 (12.7348, 1.408) -> (12.6332, 1.408) centre (12.684, 1.408) ccw
  arc A3194 (12.6332, 0.392) -> (12.7348, 0.392) centre (12.684, 0.392) ccw
  line L1453 (14.684, -8.992) -> (16.716, -8.992)
  arc A3195 (16.716, -9.0428) -> (16.716, -8.9412) centre (16.716, -8.992) ccw
  arc A3196 (14.684, -8.9412) -> (14.684, -9.0428) centre (14.684, -8.992) ccw
  line L1454 (16.716, -8.992) -> (16.716, -10.008)
  arc A3197 (16.6652, -10.008) -> (16.7668, -10.008) centre (16.716, -10.008) ccw
  arc A3198 (16.7668, -8.992) -> (16.6652, -8.992) centre (16.716, -8.992) ccw
  line L1455 (16.716, -10.008) -> (14.684, -10.008)
  arc A3199 (14.684, -9.9572) -> (14.684, -10.0588) centre (14.684, -10.008) ccw
  arc A3200 (16.716, -10.0588) -> (16.716, -9.9572) centre (16.716, -10.008) ccw
  line L1456 (14.684, -10.008) -> (14.684, -8.992)
  arc A3201 (14.7348, -8.992) -> (14.6332, -8.992) centre (14.684, -8.992) ccw
  arc A3202 (14.6332, -10.008) -> (14.7348, -10.008) centre (14.684, -10.008) ccw
  line L1457 (20.916, -10.008) -> (18.884, -10.008)
  arc A3203 (18.884, -9.9572) -> (18.884, -10.0588) centre (18.884, -10.008) ccw
  arc A3204 (20.916, -10.0588) -> (20.916, -9.9572) centre (20.916, -10.008) ccw
  line L1458 (18.884, -10.008) -> (18.884, -8.992)
  arc A3205 (18.9348, -8.992) -> (18.8332, -8.992) centre (18.884, -8.992) ccw
  arc A3206 (18.8332, -10.008) -> (18.9348, -10.008) centre (18.884, -10.008) ccw
  line L1459 (18.884, -8.992) -> (20.916, -8.992)
  arc A3207 (20.916, -9.0428) -> (20.916, -8.9412) centre (20.916, -8.992) ccw
  arc A3208 (18.884, -8.9412) -> (18.884, -9.0428) centre (18.884, -8.992) ccw
  line L1460 (20.916, -8.992) -> (20.916, -10.008)
  arc A3209 (20.8652, -10.008) -> (20.9668, -10.008) centre (20.916, -10.008) ccw
  arc A3210 (20.9668, -8.992) -> (20.8652, -8.992) centre (20.916, -8.992) ccw
  line L1461 (16.684, -8.992) -> (18.716, -8.992)
  arc A3211 (18.716, -9.0428) -> (18.716, -8.9412) centre (18.716, -8.992) ccw
  arc A3212 (16.684, -8.9412) -> (16.684, -9.0428) centre (16.684, -8.992) ccw
  line L1462 (18.716, -8.992) -> (18.716, -10.008)
  arc A3213 (18.6652, -10.008) -> (18.7668, -10.008) centre (18.716, -10.008) ccw
  arc A3214 (18.7668, -8.992) -> (18.6652, -8.992) centre (18.716, -8.992) ccw
  line L1463 (18.716, -10.008) -> (16.684, -10.008)
  arc A3215 (16.684, -9.9572) -> (16.684, -10.0588) centre (16.684, -10.008) ccw
  arc A3216 (18.716, -10.0588) -> (18.716, -9.9572) centre (18.716, -10.008) ccw
  line L1464 (16.684, -10.008) -> (16.684, -8.992)
  arc A3217 (16.7348, -8.992) -> (16.6332, -8.992) centre (16.684, -8.992) ccw
  arc A3218 (16.6332, -10.008) -> (16.7348, -10.008) centre (16.684, -10.008) ccw
  line L1465 (18.716, -15.008) -> (16.684, -15.008)
  arc A3219 (16.684, -14.9572) -> (16.684, -15.0588) centre (16.684, -15.008) ccw
  arc A3220 (18.716, -15.0588) -> (18.716, -14.9572) centre (18.716, -15.008) ccw
  line L1466 (16.684, -15.008) -> (16.684, -13.992)
  arc A3221 (16.7348, -13.992) -> (16.6332, -13.992) centre (16.684, -13.992) ccw
  arc A3222 (16.6332, -15.008) -> (16.7348, -15.008) centre (16.684, -15.008) ccw
  line L1467 (16.684, -13.992) -> (18.716, -13.992)
  arc A3223 (18.716, -14.0428) -> (18.716, -13.9412) centre (18.716, -13.992) ccw
  arc A3224 (16.684, -13.9412) -> (16.684, -14.0428) centre (16.684, -13.992) ccw
  line L1468 (18.716, -13.992) -> (18.716, -15.008)
  arc A3225 (18.6652, -15.008) -> (18.7668, -15.008) centre (18.716, -15.008) ccw
  arc A3226 (18.7668, -13.992) -> (18.6652, -13.992) centre (18.716, -13.992) ccw
  line L1469 (9.116, -24.808) -> (7.084, -24.808)
  arc A3227 (7.084, -24.7572) -> (7.084, -24.8588) centre (7.084, -24.808) ccw
  arc A3228 (9.116, -24.8588) -> (9.116, -24.7572) centre (9.116, -24.808) ccw
  line L1470 (7.084, -24.808) -> (7.084, -23.792)
  arc A3229 (7.1348, -23.792) -> (7.0332, -23.792) centre (7.084, -23.792) ccw
  arc A3230 (7.0332, -24.808) -> (7.1348, -24.808) centre (7.084, -24.808) ccw
  line L1471 (7.084, -23.792) -> (9.116, -23.792)
  arc A3231 (9.116, -23.8428) -> (9.116, -23.7412) centre (9.116, -23.792) ccw
  arc A3232 (7.084, -23.7412) -> (7.084, -23.8428) centre (7.084, -23.792) ccw
  line L1472 (9.116, -23.792) -> (9.116, -24.808)
  arc A3233 (9.0652, -24.808) -> (9.1668, -24.808) centre (9.116, -24.808) ccw
  arc A3234 (9.1668, -23.792) -> (9.0652, -23.792) centre (9.116, -23.792) ccw
  line L1473 (4.916, -24.808) -> (2.884, -24.808)
  arc A3235 (2.884, -24.7572) -> (2.884, -24.8588) centre (2.884, -24.808) ccw
  arc A3236 (4.916, -24.8588) -> (4.916, -24.7572) centre (4.916, -24.808) ccw
  line L1474 (2.884, -24.808) -> (2.884, -23.792)
  arc A3237 (2.9348, -23.792) -> (2.8332, -23.792) centre (2.884, -23.792) ccw
  arc A3238 (2.8332, -24.808) -> (2.9348, -24.808) centre (2.884, -24.808) ccw
  line L1475 (2.884, -23.792) -> (4.916, -23.792)
  arc A3239 (4.916, -23.8428) -> (4.916, -23.7412) centre (4.916, -23.792) ccw
  arc A3240 (2.884, -23.7412) -> (2.884, -23.8428) centre (2.884, -23.792) ccw
  line L1476 (4.916, -23.792) -> (4.916, -24.808)
  arc A3241 (4.8652, -24.808) -> (4.9668, -24.808) centre (4.916, -24.808) ccw
  arc A3242 (4.9668, -23.792) -> (4.8652, -23.792) centre (4.916, -23.792) ccw
  line L1477 (7.116, -24.808) -> (5.084, -24.808)
  arc A3243 (5.084, -24.7572) -> (5.084, -24.8588) centre (5.084, -24.808) ccw
  arc A3244 (7.116, -24.8588) -> (7.116, -24.7572) centre (7.116, -24.808) ccw
  line L1478 (5.084, -24.808) -> (5.084, -23.792)
  arc A3245 (5.1348, -23.792) -> (5.0332, -23.792) centre (5.084, -23.792) ccw
  arc A3246 (5.0332, -24.808) -> (5.1348, -24.808) centre (5.084, -24.808) ccw
  line L1479 (5.084, -23.792) -> (7.116, -23.792)
  arc A3247 (7.116, -23.8428) -> (7.116, -23.7412) centre (7.116, -23.792) ccw
  arc A3248 (5.084, -23.7412) -> (5.084, -23.8428) centre (5.084, -23.792) ccw
  line L1480 (7.116, -23.792) -> (7.116, -24.808)
  arc A3249 (7.0652, -24.808) -> (7.1668, -24.808) centre (7.116, -24.808) ccw
  arc A3250 (7.1668, -23.792) -> (7.0652, -23.792) centre (7.116, -23.792) ccw
  line L1481 (7.084, -13.792) -> (9.116, -13.792)
  arc A3251 (9.116, -13.8428) -> (9.116, -13.7412) centre (9.116, -13.792) ccw
  arc A3252 (7.084, -13.7412) -> (7.084, -13.8428) centre (7.084, -13.792) ccw
  line L1482 (9.116, -13.792) -> (9.116, -14.808)
  arc A3253 (9.0652, -14.808) -> (9.1668, -14.808) centre (9.116, -14.808) ccw
  arc A3254 (9.1668, -13.792) -> (9.0652, -13.792) centre (9.116, -13.792) ccw
  line L1483 (9.116, -14.808) -> (7.084, -14.808)
  arc A3255 (7.084, -14.7572) -> (7.084, -14.8588) centre (7.084, -14.808) ccw
  arc A3256 (9.116, -14.8588) -> (9.116, -14.7572) centre (9.116, -14.808) ccw
  line L1484 (7.084, -14.808) -> (7.084, -13.792)
  arc A3257 (7.1348, -13.792) -> (7.0332, -13.792) centre (7.084, -13.792) ccw
  arc A3258 (7.0332, -14.808) -> (7.1348, -14.808) centre (7.084, -14.808) ccw
  line L1485 (11.116, -24.808) -> (9.084, -24.808)
  arc A3259 (9.084, -24.7572) -> (9.084, -24.8588) centre (9.084, -24.808) ccw
  arc A3260 (11.116, -24.8588) -> (11.116, -24.7572) centre (11.116, -24.808) ccw
  line L1486 (9.084, -24.808) -> (9.084, -23.792)
  arc A3261 (9.1348, -23.792) -> (9.0332, -23.792) centre (9.084, -23.792) ccw
  arc A3262 (9.0332, -24.808) -> (9.1348, -24.808) centre (9.084, -24.808) ccw
  line L1487 (9.084, -23.792) -> (11.116, -23.792)
  arc A3263 (11.116, -23.8428) -> (11.116, -23.7412) centre (11.116, -23.792) ccw
  arc A3264 (9.084, -23.7412) -> (9.084, -23.8428) centre (9.084, -23.792) ccw
  line L1488 (11.116, -23.792) -> (11.116, -24.808)
  arc A3265 (11.0652, -24.808) -> (11.1668, -24.808) centre (11.116, -24.808) ccw
  arc A3266 (11.1668, -23.792) -> (11.0652, -23.792) centre (11.116, -23.792) ccw
  line L1489 (68.816, 37.092) -> (66.784, 37.092)
  arc A3267 (66.784, 37.1428) -> (66.784, 37.0412) centre (66.784, 37.092) ccw
  arc A3268 (68.816, 37.0412) -> (68.816, 37.1428) centre (68.816, 37.092) ccw
  line L1490 (66.784, 37.092) -> (66.784, 38.108)
  arc A3269 (66.8348, 38.108) -> (66.7332, 38.108) centre (66.784, 38.108) ccw
  arc A3270 (66.7332, 37.092) -> (66.8348, 37.092) centre (66.784, 37.092) ccw
  line L1491 (66.784, 38.108) -> (68.816, 38.108)
  arc A3271 (68.816, 38.0572) -> (68.816, 38.1588) centre (68.816, 38.108) ccw
  arc A3272 (66.784, 38.1588) -> (66.784, 38.0572) centre (66.784, 38.108) ccw
  line L1492 (68.816, 38.108) -> (68.816, 37.092)
  arc A3273 (68.7652, 37.092) -> (68.8668, 37.092) centre (68.816, 37.092) ccw
  arc A3274 (68.8668, 38.108) -> (68.7652, 38.108) centre (68.816, 38.108) ccw
  line L1493 (68.816, 36.092) -> (66.784, 36.092)
  arc A3275 (66.784, 36.1428) -> (66.784, 36.0412) centre (66.784, 36.092) ccw
  arc A3276 (68.816, 36.0412) -> (68.816, 36.1428) centre (68.816, 36.092) ccw
  line L1494 (66.784, 36.092) -> (66.784, 37.108)
  arc A3277 (66.8348, 37.108) -> (66.7332, 37.108) centre (66.784, 37.108) ccw
  arc A3278 (66.7332, 36.092) -> (66.8348, 36.092) centre (66.784, 36.092) ccw
  line L1495 (66.784, 37.108) -> (68.816, 37.108)
  arc A3279 (68.816, 37.0572) -> (68.816, 37.1588) centre (68.816, 37.108) ccw
  arc A3280 (66.784, 37.1588) -> (66.784, 37.0572) centre (66.784, 37.108) ccw
  line L1496 (68.816, 37.108) -> (68.816, 36.092)
  arc A3281 (68.7652, 36.092) -> (68.8668, 36.092) centre (68.816, 36.092) ccw
  arc A3282 (68.8668, 37.108) -> (68.7652, 37.108) centre (68.816, 37.108) ccw
  line L1497 (-27.442, 51.6) -> (-19.442, 51.6)
  arc A3283 (-19.442, 51.575) -> (-19.442, 51.625) centre (-19.442, 51.6) ccw
  arc A3284 (-27.442, 51.625) -> (-27.442, 51.575) centre (-27.442, 51.6) ccw
  line L1498 (-27.442, 59.6) -> (-19.442, 59.6)
  arc A3285 (-19.442, 59.575) -> (-19.442, 59.625) centre (-19.442, 59.6) ccw
  arc A3286 (-27.442, 59.625) -> (-27.442, 59.575) centre (-27.442, 59.6) ccw
  line L1499 (-19.442, 59.6) -> (-19.442, 51.6)
  arc A3287 (-19.467, 51.6) -> (-19.417, 51.6) centre (-19.442, 51.6) ccw
  arc A3288 (-19.417, 59.6) -> (-19.467, 59.6) centre (-19.442, 59.6) ccw
  line L1500 (25.453, -102.559) -> (19.347, -102.559)
  arc A3289 (19.347, -102.509) -> (19.347, -102.609) centre (19.347, -102.559) ccw
  arc A3290 (25.453, -102.609) -> (25.453, -102.509) centre (25.453, -102.559) ccw
  line L1501 (19.347, -102.559) -> (19.347, -110.241)
  arc A3291 (19.297, -110.241) -> (19.397, -110.241) centre (19.347, -110.241) ccw
  arc A3292 (19.397, -102.559) -> (19.297, -102.559) centre (19.347, -102.559) ccw
  line L1502 (19.347, -110.241) -> (25.453, -110.241)
  arc A3293 (25.453, -110.291) -> (25.453, -110.191) centre (25.453, -110.241) ccw
  arc A3294 (19.347, -110.191) -> (19.347, -110.291) centre (19.347, -110.241) ccw
  line L1503 (25.453, -110.241) -> (25.453, -102.559)
  arc A3295 (25.503, -102.559) -> (25.403, -102.559) centre (25.453, -102.559) ccw
  arc A3296 (25.403, -110.241) -> (25.503, -110.241) centre (25.453, -110.241) ccw
  line L1504 (24.3828, -103.5864) -> (24.0693, -103.2729)
  arc A3297 (24.0828, -103.2594) -> (24.0558, -103.2864) centre (24.0693, -103.2729) ccw
  arc A3298 (24.3694, -103.5999) -> (24.3963, -103.5729) centre (24.3828, -103.5864) ccw
  line L1505 (24.0693, -103.2729) -> (25.0099, -103.2729)
  arc A3299 (25.0099, -103.2919) -> (25.0099, -103.2538) centre (25.0099, -103.2729) ccw
  arc A3300 (24.0693, -103.2538) -> (24.0693, -103.2919) centre (24.0693, -103.2729) ccw
  line L1506 (25.0099, -103.5864) -> (25.0099, -102.9593)
  arc A3301 (25.0289, -102.9593) -> (24.9909, -102.9593) centre (25.0099, -102.9593) ccw
  arc A3302 (24.9909, -103.5864) -> (25.0289, -103.5864) centre (25.0099, -103.5864) ccw
  line L1507 (-8.524, -19.453) -> (-8.524, -13.347)
  arc A3303 (-8.474, -13.347) -> (-8.574, -13.347) centre (-8.524, -13.347) ccw
  arc A3304 (-8.574, -19.453) -> (-8.474, -19.453) centre (-8.524, -19.453) ccw
  line L1508 (-8.524, -13.347) -> (-17.476, -13.347)
  arc A3305 (-17.476, -13.297) -> (-17.476, -13.397) centre (-17.476, -13.347) ccw
  arc A3306 (-8.524, -13.397) -> (-8.524, -13.297) centre (-8.524, -13.347) ccw
  line L1509 (-17.476, -13.347) -> (-17.476, -19.453)
  arc A3307 (-17.526, -19.453) -> (-17.426, -19.453) centre (-17.476, -19.453) ccw
  arc A3308 (-17.426, -13.347) -> (-17.526, -13.347) centre (-17.476, -13.347) ccw
  line L1510 (-17.476, -19.453) -> (-8.524, -19.453)
  arc A3309 (-8.524, -19.503) -> (-8.524, -19.403) centre (-8.524, -19.453) ccw
  arc A3310 (-17.476, -19.403) -> (-17.476, -19.503) centre (-17.476, -19.453) ccw
  line L1511 (-9.5514, -18.3828) -> (-9.2379, -18.0693)
  arc A3311 (-9.2244, -18.0828) -> (-9.2514, -18.0558) centre (-9.2379, -18.0693) ccw
  arc A3312 (-9.5649, -18.3694) -> (-9.5379, -18.3963) centre (-9.5514, -18.3829) ccw
  line L1512 (-9.2379, -18.0693) -> (-9.2379, -19.0099)
  arc A3313 (-9.2569, -19.0099) -> (-9.2188, -19.0099) centre (-9.2379, -19.0099) ccw
  arc A3314 (-9.2188, -18.0693) -> (-9.2569, -18.0693) centre (-9.2379, -18.0693) ccw
  line L1513 (-9.5514, -19.0099) -> (-8.9243, -19.0099)
  arc A3315 (-8.9243, -19.0289) -> (-8.9243, -18.9909) centre (-8.9243, -19.0099) ccw
  arc A3316 (-9.5514, -18.9909) -> (-9.5514, -19.0289) centre (-9.5514, -19.0099) ccw
  line L1514 (19.047, -53.541) -> (25.153, -53.541)
  arc A3317 (25.153, -53.591) -> (25.153, -53.491) centre (25.153, -53.541) ccw
  arc A3318 (19.047, -53.491) -> (19.047, -53.591) centre (19.047, -53.541) ccw
  line L1515 (25.153, -53.541) -> (25.153, -45.859)
  arc A3319 (25.203, -45.859) -> (25.103, -45.859) centre (25.153, -45.859) ccw
  arc A3320 (25.103, -53.541) -> (25.203, -53.541) centre (25.153, -53.541) ccw
  line L1516 (25.153, -45.859) -> (19.047, -45.859)
  arc A3321 (19.047, -45.809) -> (19.047, -45.909) centre (19.047, -45.859) ccw
  arc A3322 (25.153, -45.909) -> (25.153, -45.809) centre (25.153, -45.859) ccw
  line L1517 (19.047, -45.859) -> (19.047, -53.541)
  arc A3323 (18.997, -53.541) -> (19.097, -53.541) centre (19.047, -53.541) ccw
  arc A3324 (19.097, -45.859) -> (18.997, -45.859) centre (19.047, -45.859) ccw
  line L1518 (19.8028, -53.3729) -> (19.4893, -53.0594)
  arc A3325 (19.5028, -53.0459) -> (19.4758, -53.0728) centre (19.4893, -53.0594) ccw
  arc A3326 (19.7894, -53.3864) -> (19.8163, -53.3594) centre (19.8028, -53.3729) ccw
  line L1519 (19.4893, -53.0594) -> (20.4299, -53.0594)
  arc A3327 (20.4299, -53.0784) -> (20.4299, -53.0403) centre (20.4299, -53.0594) ccw
  arc A3328 (19.4893, -53.0403) -> (19.4893, -53.0784) centre (19.4893, -53.0594) ccw
  line L1520 (20.4299, -53.3729) -> (20.4299, -52.7458)
  arc A3329 (20.4489, -52.7458) -> (20.4109, -52.7458) centre (20.4299, -52.7458) ccw
  arc A3330 (20.4109, -53.3729) -> (20.4489, -53.3729) centre (20.4299, -53.3729) ccw
  line L1521 (-33.24, -43.1) -> (-37.56, -43.1)
  arc A3331 (-37.56, -43.0619) -> (-37.56, -43.1381) centre (-37.56, -43.1) ccw
  arc A3332 (-33.24, -43.1381) -> (-33.24, -43.0619) centre (-33.24, -43.1) ccw
  line L1522 (-37.56, -40.5) -> (-33.24, -40.5)
  arc A3333 (-33.24, -40.5381) -> (-33.24, -40.4619) centre (-33.24, -40.5) ccw
  arc A3334 (-37.56, -40.4619) -> (-37.56, -40.5381) centre (-37.56, -40.5) ccw
  line L1523 (-33.24, -54.7) -> (-37.56, -54.7)
  arc A3335 (-37.56, -54.6619) -> (-37.56, -54.7381) centre (-37.56, -54.7) ccw
  arc A3336 (-33.24, -54.7381) -> (-33.24, -54.6619) centre (-33.24, -54.7) ccw
  line L1524 (-37.56, -52.1) -> (-33.24, -52.1)
  arc A3337 (-33.24, -52.1381) -> (-33.24, -52.0619) centre (-33.24, -52.1) ccw
  arc A3338 (-37.56, -52.0619) -> (-37.56, -52.1381) centre (-37.56, -52.1) ccw
  line L1525 (-60.925, -51) -> (-59.675, -51)
  arc A3339 (-59.675, -51.0317) -> (-59.675, -50.9682) centre (-59.675, -51) ccw
  arc A3340 (-60.925, -50.9682) -> (-60.925, -51.0317) centre (-60.925, -51) ccw
  line L1526 (-59.675, -49) -> (-60.925, -49)
  arc A3341 (-60.925, -48.9682) -> (-60.925, -49.0317) centre (-60.925, -49) ccw
  arc A3342 (-59.675, -49.0317) -> (-59.675, -48.9682) centre (-59.675, -49) ccw
  line L1527 (-60.925, -49) -> (-60.925, -51)
  arc A3343 (-60.9567, -51) -> (-60.8933, -51) centre (-60.925, -51) ccw
  arc A3344 (-60.8933, -49) -> (-60.9567, -49) centre (-60.925, -49) ccw
  line L1528 (-59.675, -51) -> (-59.675, -49)
  arc A3345 (-59.6433, -49) -> (-59.7067, -49) centre (-59.675, -49) ccw
  arc A3346 (-59.7067, -51) -> (-59.6433, -51) centre (-59.675, -51) ccw
  line L1529 (-60.925, -47.4) -> (-59.675, -47.4)
  arc A3347 (-59.675, -47.4317) -> (-59.675, -47.3682) centre (-59.675, -47.4) ccw
  arc A3348 (-60.925, -47.3682) -> (-60.925, -47.4317) centre (-60.925, -47.4) ccw
  line L1530 (-59.675, -45.4) -> (-60.925, -45.4)
  arc A3349 (-60.925, -45.3682) -> (-60.925, -45.4317) centre (-60.925, -45.4) ccw
  arc A3350 (-59.675, -45.4317) -> (-59.675, -45.3682) centre (-59.675, -45.4) ccw
  line L1531 (-60.925, -45.4) -> (-60.925, -47.4)
  arc A3351 (-60.9567, -47.4) -> (-60.8933, -47.4) centre (-60.925, -47.4) ccw
  arc A3352 (-60.8933, -45.4) -> (-60.9567, -45.4) centre (-60.925, -45.4) ccw
  line L1532 (-59.675, -47.4) -> (-59.675, -45.4)
  arc A3353 (-59.6433, -45.4) -> (-59.7067, -45.4) centre (-59.675, -45.4) ccw
  arc A3354 (-59.7067, -47.4) -> (-59.6433, -47.4) centre (-59.675, -47.4) ccw
  line L1533 (-45.078, -35.44) -> (-45.078, -36.76)
  arc A3355 (-45.1161, -36.76) -> (-45.0399, -36.76) centre (-45.078, -36.76) ccw
  arc A3356 (-45.0399, -35.44) -> (-45.1161, -35.44) centre (-45.078, -35.44) ccw
  line L1534 (-45.078, -36.76) -> (-47.922, -36.76)
  arc A3357 (-47.922, -36.7219) -> (-47.922, -36.7981) centre (-47.922, -36.76) ccw
  arc A3358 (-45.078, -36.7981) -> (-45.078, -36.7219) centre (-45.078, -36.76) ccw
  line L1535 (-47.922, -36.76) -> (-47.922, -35.44)
  arc A3359 (-47.8839, -35.44) -> (-47.9601, -35.44) centre (-47.922, -35.44) ccw
  arc A3360 (-47.9601, -36.76) -> (-47.8839, -36.76) centre (-47.922, -36.76) ccw
  line L1536 (-47.922, -35.44) -> (-45.078, -35.44)
  arc A3361 (-45.078, -35.4781) -> (-45.078, -35.4019) centre (-45.078, -35.44) ccw
  arc A3362 (-47.922, -35.4019) -> (-47.922, -35.4781) centre (-47.922, -35.44) ccw
  line L1537 (-53.578, -35.44) -> (-53.578, -36.76)
  arc A3363 (-53.6161, -36.76) -> (-53.5399, -36.76) centre (-53.578, -36.76) ccw
  arc A3364 (-53.5399, -35.44) -> (-53.6161, -35.44) centre (-53.578, -35.44) ccw
  line L1538 (-53.578, -36.76) -> (-56.422, -36.76)
  arc A3365 (-56.422, -36.7219) -> (-56.422, -36.7981) centre (-56.422, -36.76) ccw
  arc A3366 (-53.578, -36.7981) -> (-53.578, -36.7219) centre (-53.578, -36.76) ccw
  line L1539 (-56.422, -36.76) -> (-56.422, -35.44)
  arc A3367 (-56.3839, -35.44) -> (-56.4601, -35.44) centre (-56.422, -35.44) ccw
  arc A3368 (-56.4601, -36.76) -> (-56.3839, -36.76) centre (-56.422, -36.76) ccw
  line L1540 (-56.422, -35.44) -> (-53.578, -35.44)
  arc A3369 (-53.578, -35.4781) -> (-53.578, -35.4019) centre (-53.578, -35.44) ccw
  arc A3370 (-56.422, -35.4019) -> (-56.422, -35.4781) centre (-56.422, -35.44) ccw
  line L1541 (-50.278, -35.44) -> (-50.278, -36.76)
  arc A3371 (-50.3161, -36.76) -> (-50.2399, -36.76) centre (-50.278, -36.76) ccw
  arc A3372 (-50.2399, -35.44) -> (-50.3161, -35.44) centre (-50.278, -35.44) ccw
  line L1542 (-50.278, -36.76) -> (-53.122, -36.76)
  arc A3373 (-53.122, -36.7219) -> (-53.122, -36.7981) centre (-53.122, -36.76) ccw
  arc A3374 (-50.278, -36.7981) -> (-50.278, -36.7219) centre (-50.278, -36.76) ccw
  line L1543 (-53.122, -36.76) -> (-53.122, -35.44)
  arc A3375 (-53.0839, -35.44) -> (-53.1601, -35.44) centre (-53.122, -35.44) ccw
  arc A3376 (-53.1601, -36.76) -> (-53.0839, -36.76) centre (-53.122, -36.76) ccw
  line L1544 (-53.122, -35.44) -> (-50.278, -35.44)
  arc A3377 (-50.278, -35.4781) -> (-50.278, -35.4019) centre (-50.278, -35.44) ccw
  arc A3378 (-53.122, -35.4019) -> (-53.122, -35.4781) centre (-53.122, -35.44) ccw
  line L1545 (-37.35, -37.75) -> (-33.45, -37.75)
  arc A3379 (-33.45, -37.7817) -> (-33.45, -37.7182) centre (-33.45, -37.75) ccw
  arc A3380 (-37.35, -37.7182) -> (-37.35, -37.7817) centre (-37.35, -37.75) ccw
  line L1546 (-33.45, -40.25) -> (-37.35, -40.25)
  arc A3381 (-37.35, -40.2182) -> (-37.35, -40.2817) centre (-37.35, -40.25) ccw
  arc A3382 (-33.45, -40.2817) -> (-33.45, -40.2182) centre (-33.45, -40.25) ccw
  line L1547 (-37.35, -54.95) -> (-33.45, -54.95)
  arc A3383 (-33.45, -54.9817) -> (-33.45, -54.9182) centre (-33.45, -54.95) ccw
  arc A3384 (-37.35, -54.9182) -> (-37.35, -54.9817) centre (-37.35, -54.95) ccw
  line L1548 (-33.45, -57.45) -> (-37.35, -57.45)
  arc A3385 (-37.35, -57.4182) -> (-37.35, -57.4817) centre (-37.35, -57.45) ccw
  arc A3386 (-33.45, -57.4817) -> (-33.45, -57.4182) centre (-33.45, -57.45) ccw
  line L1549 (-48.222, -59.96) -> (-48.222, -58.64)
  arc A3387 (-48.1839, -58.64) -> (-48.2601, -58.64) centre (-48.222, -58.64) ccw
  arc A3388 (-48.2601, -59.96) -> (-48.1839, -59.96) centre (-48.222, -59.96) ccw
  line L1550 (-48.222, -58.64) -> (-45.378, -58.64)
  arc A3389 (-45.378, -58.6781) -> (-45.378, -58.6019) centre (-45.378, -58.64) ccw
  arc A3390 (-48.222, -58.6019) -> (-48.222, -58.6781) centre (-48.222, -58.64) ccw
  line L1551 (-45.378, -58.64) -> (-45.378, -59.96)
  arc A3391 (-45.4161, -59.96) -> (-45.3399, -59.96) centre (-45.378, -59.96) ccw
  arc A3392 (-45.3399, -58.64) -> (-45.4161, -58.64) centre (-45.378, -58.64) ccw
  line L1552 (-45.378, -59.96) -> (-48.222, -59.96)
  arc A3393 (-48.222, -59.9219) -> (-48.222, -59.9981) centre (-48.222, -59.96) ccw
  arc A3394 (-45.378, -59.9981) -> (-45.378, -59.9219) centre (-45.378, -59.96) ccw
  line L1553 (-51.622, -59.96) -> (-51.622, -58.64)
  arc A3395 (-51.5839, -58.64) -> (-51.6601, -58.64) centre (-51.622, -58.64) ccw
  arc A3396 (-51.6601, -59.96) -> (-51.5839, -59.96) centre (-51.622, -59.96) ccw
  line L1554 (-51.622, -58.64) -> (-48.778, -58.64)
  arc A3397 (-48.778, -58.6781) -> (-48.778, -58.6019) centre (-48.778, -58.64) ccw
  arc A3398 (-51.622, -58.6019) -> (-51.622, -58.6781) centre (-51.622, -58.64) ccw
  line L1555 (-48.778, -58.64) -> (-48.778, -59.96)
  arc A3399 (-48.8161, -59.96) -> (-48.7399, -59.96) centre (-48.778, -59.96) ccw
  arc A3400 (-48.7399, -58.64) -> (-48.8161, -58.64) centre (-48.778, -58.64) ccw
  line L1556 (-48.778, -59.96) -> (-51.622, -59.96)
  arc A3401 (-51.622, -59.9219) -> (-51.622, -59.9981) centre (-51.622, -59.96) ccw
  arc A3402 (-48.778, -59.9981) -> (-48.778, -59.9219) centre (-48.778, -59.96) ccw
  line L1557 (-55.022, -59.96) -> (-55.022, -58.64)
  arc A3403 (-54.9839, -58.64) -> (-55.0601, -58.64) centre (-55.022, -58.64) ccw
  arc A3404 (-55.0601, -59.96) -> (-54.9839, -59.96) centre (-55.022, -59.96) ccw
  line L1558 (-55.022, -58.64) -> (-52.178, -58.64)